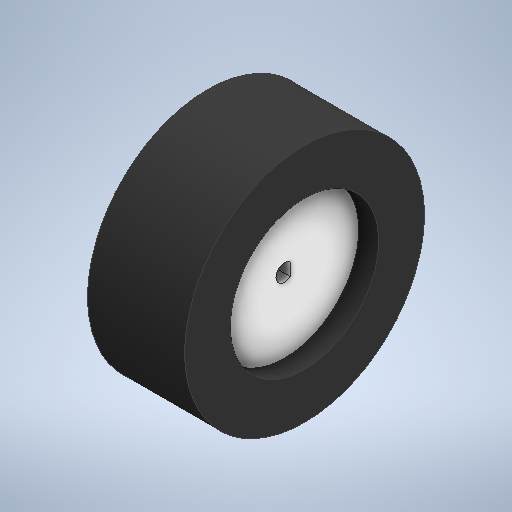
# Autodesk Inventor part: llanta
Saved by Autodesk Inventor 2025.2 (Build 292293000, 293)
## iProperties
Created: 2025-06-11
Part Number: llanta
Material: Generic
Document SubType Name: Modeling
Designer: cdavi
Density: 1 g/cm^3
Appearance: Default
Author: cdavi
Autodesk Inventor part; units mm, degrees
ref_plane "YZ Plane" through (0, 0, 0) normal (1, 0, 0) x (0, 1, 0)
ref_plane "XZ Plane" through (0, 0, 0) normal (0, 1, 0) x (-1, 0, 0)
ref_plane "XY Plane" through (0, 0, 0) normal (0, 0, 1) x (1, 0, 0)
sketch "Sketch1" plane through (0, 0, 0) normal (1, 0, 0) x (0, 1, 0)
  circle A0 centre (0, 0) radius 21
  circle A1 centre (0, 0) radius 13
  dimension "d0" = 42
  dimension "d1" = 8
  constraints: 2 centre point, 2 coincident
  measures "d0" diameter of A0
  measures "d1" radial gap between concentric circles of A1 A0
extrude "Extrusion1" add sketch "Sketch1" along normal blind 17
extrude "Extrusion2" add sketch "Sketch1" along normal blind 13.5 separate body contours A1
sketch "Sketch2" plane through (0, 0, 0) normal (-1, 0, 0) x (0, 0, 1)
  circle A0 centre (0, 0) radius 10
  circle A1 centre (0, 0) radius 12
  circle A2 centre (0, 0) radius 13 projected
  line L0 (0, 0) -> (2.0838, 11.8177) construction
  line L1 (0, 0) -> (0, 12)
  line L2 (0, 0) -> (-2.0838, 11.8177) construction
  line L3 (-2.0838, 11.8177) -> (-1.7365, 9.8481)
  line L4 (1.7365, 9.8481) -> (2.0838, 11.8177)
  line L5 (-3.4202, 9.3969) -> (-4.1042, 11.2763)
  line L6 (-7.7135, 9.1925) -> (-6.4279, 7.6604)
  line L7 (-7.6604, 6.4279) -> (-9.1925, 7.7135)
  line L8 (-11.2763, 4.1042) -> (-9.3969, 3.4202)
  line L9 (-9.8481, 1.7365) -> (-11.8177, 2.0838)
  line L10 (-11.8177, -2.0838) -> (-9.8481, -1.7365)
  line L11 (-9.3969, -3.4202) -> (-11.2763, -4.1042)
  line L12 (-9.1925, -7.7135) -> (-7.6604, -6.4279)
  line L13 (-6.4279, -7.6604) -> (-7.7135, -9.1925)
  line L14 (-4.1042, -11.2763) -> (-3.4202, -9.3969)
  line L15 (-1.7365, -9.8481) -> (-2.0838, -11.8177)
  line L16 (2.0838, -11.8177) -> (1.7365, -9.8481)
  line L17 (3.4202, -9.3969) -> (4.1042, -11.2763)
  line L18 (7.7135, -9.1925) -> (6.4279, -7.6604)
  line L19 (7.6604, -6.4279) -> (9.1925, -7.7135)
  line L20 (11.2763, -4.1042) -> (9.3969, -3.4202)
  line L21 (9.8481, -1.7365) -> (11.8177, -2.0838)
  line L22 (11.8177, 2.0838) -> (9.8481, 1.7365)
  line L23 (9.3969, 3.4202) -> (11.2763, 4.1042)
  line L24 (9.1925, 7.7135) -> (7.6604, 6.4279)
  line L25 (6.4279, 7.6604) -> (7.7135, 9.1925)
  line L26 (4.1042, 11.2763) -> (3.4202, 9.3969)
  dimension "d7" = 2
  dimension "d6" = 1
  dimension "d8" = 10
  dimension "d9" = 3.473
  dimension "d12" = 360
  constraints: 54 end point, 2 coincident, 2 point on line, 1 collinear, 1 symmetric about line, 1 vertical, 81 other
  measures "d8" angle of L1 L0
  measures "d9" distance of L4.start L3.end
extrude "Extrusion3" cut sketch "Sketch2" against normal blind 8 contours A0 | A0 L23 A1 L22 | L21 A1 L20 A0 | A0 L25 A1 L24 | L19 A1 L18 A0 | A0 L4 A1 L26 | L17 A1 L16 A0 | L15 A1 L14 A0 | A0 L5 A1 L3 | L13 A1 L12 A0 | A0 L7 A1 L6 | L11 A1 L10 A0 | A0 L9 A1 L8 | A2 bodies 2
sketch "Sketch3" plane through (13.5, 0, 0) normal (1, 0, 0) x (0, 0, -1)
  circle A0 centre (0, 0) radius 1.5
  line L0 (1, 1.118) -> (1, -1.118)
  dimension "d16" = 3
  dimension "d17" = 1
  constraints: 2 end point, 2 point on circle, 1 centre point, 1 coincident, 1 vertical
  measures "d16" diameter of A0
  measures "d17" distance from line of L0 A0.centre
extrude "Extrusion4" cut sketch "Sketch3" against normal through all contours L0 A0 picked at (0.1703, -0.0604) bodies 2
body "Solid1"
body "Solid2"
